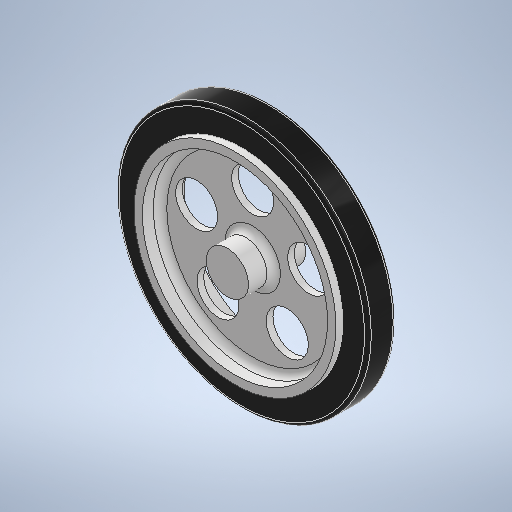
# Autodesk Inventor part: Wheel
Saved by Autodesk Inventor 2025.2 (Build 292293000, 293)
## iProperties
Created: 2025-02-25
Part Number: Wheel
Material: Generic
Document SubType Name: Modeling
Designer: Sergio Quintero
Density: 1 g/cm^3
Appearance: Default
Author: Sergio Quintero
Autodesk Inventor part; units mm, degrees
ref_plane "YZ Plane" through (0, 0, 0) normal (1, 0, 0) x (0, 1, 0)
ref_plane "XZ Plane" through (0, 0, 0) normal (0, 1, 0) x (-1, 0, 0)
ref_plane "XY Plane" through (0, 0, 0) normal (0, 0, 1) x (1, 0, 0)
sketch "Sketch1" plane through (0, 0, 0) normal (0, 0, 1) x (1, 0, 0)
  circle A0 centre (0, 0) radius 75
  circle A1 centre (0, 0) radius 60
  dimension "d0" = 150
  dimension "d1" = 120
  constraints: 2 centre point, 2 coincident
  measures "d0" diameter of A0
  measures "d1" diameter of A1
extrude "Extrusion1" add sketch "Sketch1" along normal mid plane 17
fillet "Fillet1" radius 2 2 edges at (-75, 0, 8.5) (-75, 0, -8.5)
sketch "Sketch2" plane through (0, 0, 0) normal (0, 0, 1) x (1, 0, 0)
  circle A0 centre (0, 0) radius 60
  circle A1 centre (0, 0) radius 55
  dimension "d7" = 110
  constraints: 2 centre point, 2 coincident
  measures "d7" diameter of A1
extrude "Extrusion2" add sketch "Sketch2" along normal mid plane 25 separate body
sketch "Sketch3" plane through (0, 0, 0) normal (0, 0, 1) x (1, 0, 0)
  circle A0 centre (0, 0) radius 55
  constraints: 1 centre point, 1 coincident
extrude "Extrusion3" add sketch "Sketch3" along normal mid plane 4 bodies 2
fillet "Fillet2" radius 4 1 edges at (-55, 0, -2)
sketch "Sketch4" plane through (0, 0, -2) normal (0, 0, -1) x (-1, 0, 0)
  circle A0 centre (0, 35) radius 12.5
  circle A1 centre (-33.287, 10.8156) radius 12.5
  circle A2 centre (-20.5725, -28.3156) radius 12.5
  circle A3 centre (20.5725, -28.3156) radius 12.5
  circle A4 centre (33.287, 10.8156) radius 12.5
  point P0 (0, 0)
  dimension "d11" = 25
  dimension "d12" = 35
  dimension "d15" = 360
  constraints: 5 centre point, 11 other
  measures "d11" diameter of A0
  measures "d12" distance of point (0, 0) A0.centre
extrude "Extrusion4" cut sketch "Sketch4" against normal blind 4 bodies 2
sketch "Sketch5" plane through (0, 0, -2) normal (0, 0, -1) x (-1, 0, 0)
  circle A0 centre (0, 0) radius 51 projected
  circle A1 centre (0, 0) radius 12.5
  dimension "d19" = 25
  constraints: 1 centre point, 1 coincident
  measures "d19" diameter of A1
extrude "Extrusion5" add sketch "Sketch5" along normal blind 15 contours A1 bodies 2
mirror "Mirror1" about plane through (0, 0, 0) normal (0, 0, 1) of "Extrusion5" bodies 2
fillet "Fillet3" radius 4 1 edges at (-55, 0, 2)
fillet "Fillet4" radius 4 2 edges at (12.5, 0, 2) (12.5, 0, -2)
body "Solid1"
body "Solid2"
